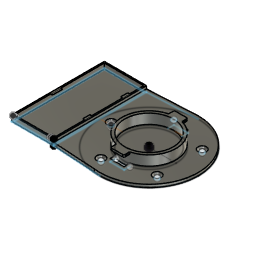
Ip Camera Mount (Autodesk Fusion 360 design; units mm, degrees)
Autodesk Fusion 360 part; units mm, degrees
sketch "Sketch1" plane through (0, 0, 0) normal (0, 0, 1) x (1, 0, 0)
  circle A0 centre (0, 0) radius 17.25
  circle A1 centre (0, 0) radius 19.25
  line L0 (0, 19.25) -> (5, 19.25) construction
  line L1 (5, 19.25) -> (-5, 19.25) construction
  line L2 (-5, 19.25) -> (-5, 22.75) construction
  line L3 (-5, 22.75) -> (5, 22.75) construction
  line L4 (5, 22.75) -> (5, 19.25) construction
  line L5 (-5, 22.75) -> (-5, 18.5893)
  line L6 (-5, 22.75) -> (5, 22.75)
  line L7 (5, 18.5893) -> (5, 22.75)
  line L8 (0, 0) -> (17.25, 0) construction
  line L9 (-5, -22.75) -> (-5, -18.5893)
  line L10 (-5, -22.75) -> (5, -22.75)
  line L11 (5, -18.5893) -> (5, -22.75)
  circle A2 centre (0, 0) radius 1.5
  circle A3 centre (0, 0) radius 35
  line L12 (-19.2494, 0.1529) -> (-34.9997, 0.1529) construction
  circle A4 centre (-27.1245, 0.1529) radius 1.5
  circle A5 centre (-8.5273, -25.7497) radius 1.5
  circle A6 centre (21.8543, -16.0671) radius 1.5
  circle A7 centre (22.0341, 15.8197) radius 1.5
  circle A8 centre (-8.2366, 25.8442) radius 1.5
  line L13 (-34.9997, 0.1529) -> (-36, 0.1529) construction
  line L14 (-36, 0.1529) -> (-36, 32.1529) construction
  line L15 (-36, 32.1529) -> (-64, 32.1529)
  line L16 (-64, 32.1529) -> (-64, -31.8471)
  line L17 (-64, -31.8471) -> (-36, -31.8471)
  line L18 (-36, -31.8471) -> (-36, 32.1529)
  line L19 (-65, 33.1529) -> (-65, -32.8471)
  line L20 (-65, -32.8471) -> (-35, -32.8471)
  line L21 (-35, -32.8471) -> (-35, 33.1529)
  line L22 (-35, 33.1529) -> (-65, 33.1529)
  line L23 (0, -35) -> (-35, -32.8471)
  line L24 (0, 35) -> (-35, 33.1529)
  dimension "d1" = 34.5
  dimension "d2" = 2
  dimension "d3" = 5
  dimension "d4" = 10
  dimension "d5" = 3.5
  dimension "d6" = 3
  dimension "d17" = 70
  dimension "d18" = 3
  dimension "d20" = 360
  dimension "d24" = 32
  dimension "d25" = 28
  dimension "d26" = 64
  dimension "d27" = 1
  constraint coincident A0.centre A1.centre
  constraint coincident A1 L0.start
  constraint horizontal L0
  constraint horizontal L1
  constraint vertical L2
  constraint horizontal L3
  constraint vertical L4
  constraint coincident A1 L5.end
  constraint perpendicular L3 L5
  constraint coincident A1 L7.start
  constraint perpendicular L6 L7
  constraint coincident A0 L8.end
  constraint horizontal L8
  constraint symmetric L2.end L8 L9.start
  constraint symmetric L3.end L8 L10.end
  constraint symmetric L5.end L8 L9.end
  constraint symmetric L7.start L8 L11.start
  constraint concentric A0 A2
  constraint coincident A1 L12.start
  constraint coincident A3 L12.end
  constraint horizontal L12
  constraint midpoint L12 A4.centre
  constraint parallel L12 L13
  constraint perpendicular L13 L14
  constraint horizontal L15
  constraint vertical L16
  constraint horizontal L17
  constraint vertical L18
  constraint coincident A3 L23.start
  constraint coincident A3 L24.start
  measures "d1" diameter of A0
  measures "d3" distance of L0.start L0.end
  measures "d4" distance of L0.end L1.end
  measures "d5" distance of L0.end L3.end
  measures "d6" diameter of A2
  measures "d17" diameter of A3
  measures "d18" diameter of A4
  measures "d24" distance of L13.end L14.end
  measures "d25" distance of L14.end L15.end
  measures "d26" distance of L14.end L17.end
extrude "Extrude1" add sketch "Sketch1" along normal blind 9 contours A1
extrude "Extrude2" add sketch "Sketch1" along normal blind 2 contours A0 | A3 L23 L24 | A3 L24 | A3 L23 | A3 L21 L24 | A3 L21 L23
extrude "Extrude3" add sketch "Sketch1" against normal blind 1.5 from surface at 9 contours A1 L5 L6 L7 | A1 L9 L10 L11
chamfer "Chamfer1" distance 0.25 angle 45 4 edges at (-5, 20.6697, 9) (5, 20.6697, 9) (5, -20.6697, 9) (-5, -20.6697, 9)
chamfer "Chamfer2" distance 0.25 angle 45 4 edges at (5, -20.6697, 7.5) (-5, -20.6697, 7.5) (-5, 20.6697, 7.5) (5, 20.6697, 7.5)
chamfer "Chamfer4" distance 1.5 angle 45 5 edges at (-28.523, 0.6953, 2) (20.6356, 16.3621, 2) (20.4559, -15.5247, 2) (-9.9258, -25.2073, 2) (-9.635, 26.3866, 2)
fillet "Fillet1" radius 1 4 edges at (5, 22.75, 8.25) (-5, 22.75, 8.25) (-5, -22.75, 8.25) (5, -22.75, 8.25)
extrude "Extrude4" add sketch "Sketch1" along normal blind 4 contours L19 L20 L21 L22
sketch "Sketch2" plane through (0, -32.8471, 0) normal (0, -1, 0) x (1, 0, 0)
  line L0 (-65, 0) -> (-35, 0)
  line L1 (-35, 0) -> (-35, 2)
  line L2 (-35, 2) -> (-35, 4)
  line L3 (-35, 4) -> (-65, 4)
  line L4 (-65, 4) -> (-65, 0)
  line L5 (-35, 4) -> (-35, 0) construction
  line L6 (-36, 3.5) -> (-37.3, 4)
  line L7 (-37.3, 4) -> (-36, 4)
  line L8 (-36, 3.5) -> (-36, 4)
  line L9 (-64, 3.5) -> (-62.7, 4)
  line L10 (-62.7, 4) -> (-64, 4)
  line L11 (-64, 3.5) -> (-64, 4)
  constraint coincident L2.end L3.start
  constraint coincident L0.end L1.start
  constraint coincident L3 L6.end
  constraint coincident L3 L7.end
  constraint perpendicular L7 L8
  constraint coincident L3 L9.end
  constraint coincident L3 L10.end
  constraint perpendicular L3 L11
extrude "Extrude5" add sketch "Sketch2" against normal blind 7 from surface at -27 contours L3 L9 L10 L11
extrude "Extrude6" add sketch "Sketch2" against normal blind 5 from surface at -23 contours L3 L6 L7 L8
extrude "Extrude8" add sketch "Sketch1" along normal blind 0.2 contours L15 L16 L17 L18
extrude "Extrude9" add sketch "Sketch2" against normal blind 5 from surface at -50 contours L3 L6 L7 L8
named bodies: "Camera mount"
